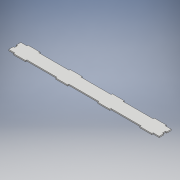
# Autodesk Inventor part: F1
Saved by Autodesk Inventor 2018 (Build 220112000, 112)
## iProperties
Created: 2018-03-06
Part Number: F1
Material: Generic
Document SubType Name: Modeling
Designer: isai
Density: 1 g/cm^3
Appearance: Default
Author: isai
Autodesk Inventor part; units mm, degrees
ref_plane "YZ Plane" through (0, 0, 0) normal (1, 0, 0) x (0, 1, 0)
ref_plane "XZ Plane" through (0, 0, 0) normal (0, 1, 0) x (-1, 0, 0)
sketch "Sketch1" plane through (0, 0, 0) normal (0, 0, 1) x (1, 0, 0)
  line L0 (29, 29) -> (9, 29)
  line L1 (9, 29) -> (9, 25)
  line L2 (9, 25) -> (-31, 25)
  line L3 (-31, 25) -> (-31, 29)
  line L4 (-31, 29) -> (-130.3333, 29)
  line L5 (-130.3333, 29) -> (-130.3333, 25)
  line L6 (-130.3333, 25) -> (-170.3333, 25)
  line L7 (-170.3333, 25) -> (-170.3333, 29)
  line L8 (-170.3333, 29) -> (-269.6667, 29)
  line L9 (-269.6667, 29) -> (-269.6667, 25)
  line L10 (-269.6667, 25) -> (-309.6667, 25)
  line L11 (-309.6667, 25) -> (-309.6667, 29)
  line L12 (-309.6667, 29) -> (-409, 29)
  line L13 (-409, 29) -> (-409, 25)
  line L14 (-409, 25) -> (-449, 25)
  line L15 (-449, 25) -> (-449, 29)
  line L16 (-449, 29) -> (-469, 29)
  line L17 (29, 29) -> (29, 69)
  line L18 (-469, 29) -> (-469, 69)
  line L19 (-469, 49) -> (-556.7501, 49)
  line L20 (9, 69) -> (9, 73)
  line L21 (9, 73) -> (-31, 73)
  line L22 (-31, 73) -> (-31, 69)
  line L23 (-130.3333, 69) -> (-130.3333, 73)
  line L24 (-130.3333, 73) -> (-170.3333, 73)
  line L25 (-409, 73) -> (-449, 73)
  line L26 (-449, 73) -> (-449, 69)
  line L27 (-409, 69) -> (-409, 73)
  line L28 (-309.6667, 73) -> (-309.6667, 69)
  line L29 (-170.3333, 73) -> (-170.3333, 69)
  line L30 (-269.6667, 69) -> (-269.6667, 73)
  line L31 (-269.6667, 73) -> (-309.6667, 73)
  line L32 (-170.3333, 69) -> (-269.6667, 69)
  line L33 (29, 69) -> (9, 69)
  line L34 (-31, 69) -> (-130.3333, 69)
  line L35 (-309.6667, 69) -> (-409, 69)
  line L36 (-449, 69) -> (-469, 69)
  point P0 (0, 0)
  dimension "d0" = 40
  dimension "d1" = 40
  dimension "d2" = 40
  dimension "d3" = 40
  dimension "d4" = 40
  dimension "d5" = 498
  dimension "d6" = 40
  constraints: 74 end point, 16 symmetric about line, 5 parallel, 1 horizontal, 1 midpoint, 1 perpendicular, 1 vertical
  measures "d0" distance of L0.start L17.end
  measures "d1" distance of L1.end L2.end
  measures "d2" distance of L5.end L6.end
  measures "d3" distance of L9.end L11.start
  measures "d4" distance of L14.start L14.end
  measures "d5" distance of L17.end L18.end
  measures "d6" distance of L16.end L18.end
extrude "Extrusion1" add sketch "Sketch1" along normal blind 4
sketch "Sketch3" plane through (0, 0, 4) normal (0, 0, 1) x (1, 0, 0)
  line L0 (9, 25) -> (9, 29) projected
  line L1 (9, 29) -> (29, 29) projected
  line L2 (29, 29) -> (29, 69) projected
  line L3 (29, 69) -> (9, 69) projected
  line L4 (9, 69) -> (9, 73) projected
  line L5 (9, 73) -> (-31, 73) projected
  line L6 (-31, 73) -> (-31, 69) projected
  line L7 (-31, 69) -> (-130.3333, 69) projected
  line L8 (-130.3333, 69) -> (-130.3333, 73) projected
  line L9 (-130.3333, 73) -> (-170.3333, 73) projected
  line L10 (-170.3333, 73) -> (-170.3333, 69) projected
  line L11 (-170.3333, 69) -> (-269.6667, 69) projected
  line L12 (-269.6667, 69) -> (-269.6667, 73) projected
  line L13 (-269.6667, 73) -> (-309.6667, 73) projected
  line L14 (-309.6667, 73) -> (-309.6667, 69) projected
  line L15 (-309.6667, 69) -> (-409, 69) projected
  line L16 (-409, 69) -> (-409, 73) projected
  line L17 (-409, 73) -> (-449, 73) projected
  line L18 (-449, 73) -> (-449, 69) projected
  line L19 (-449, 69) -> (-469, 69) projected
  line L20 (-469, 69) -> (-469, 29) projected
  line L21 (-469, 29) -> (-449, 29) projected
  line L22 (-449, 29) -> (-449, 25) projected
  line L23 (-449, 25) -> (-409, 25) projected
  line L24 (-409, 25) -> (-409, 29) projected
  line L25 (-409, 29) -> (-309.6667, 29) projected
  line L26 (-309.6667, 29) -> (-309.6667, 25) projected
  line L27 (-309.6667, 25) -> (-269.6667, 25) projected
  line L28 (-269.6667, 25) -> (-269.6667, 29) projected
  line L29 (-269.6667, 29) -> (-170.3333, 29) projected
  line L30 (-170.3333, 29) -> (-170.3333, 25) projected
  line L31 (-170.3333, 25) -> (-130.3333, 25) projected
  line L32 (-130.3333, 25) -> (-130.3333, 29) projected
  line L33 (-130.3333, 29) -> (-31, 29) projected
  line L34 (-31, 29) -> (-31, 25) projected
  line L35 (-31, 25) -> (9, 25) projected
  line L36 (-234.0151, 149.1478) -> (-234.0151, 116.0125)
  line L37 (25, 54) -> (29, 54)
  line L38 (29, 54) -> (29, 44)
  line L39 (29, 44) -> (25, 44)
  line L40 (25, 44) -> (25, 54)
  point P0 (0, 0)
  point P1 (29, 49)
  dimension "d15" = 498
  dimension "d16" = 4
  dimension "d17" = 10
  constraints: 10 end point, 2 midpoint, 2 parallel, 1 horizontal, 1 perpendicular, 1 vertical
  measures "d15" distance between parallel lines of L2 L20
  measures "d16" distance of L38.end L39.end
  measures "d17" distance of L37.end L38.end
extrude "Extrusion3" cut sketch "Sketch3" against normal blind 4 contours L39 L40 L37 L2
ref_plane "Work Plane2" through (-220, 69, 4) normal (1, 0, 0) x (0, 0, -1)
mirror "Mirror1" about plane through (-220, 69, 4) normal (1, 0, 0) of "Extrusion3"
body "Solid1"
